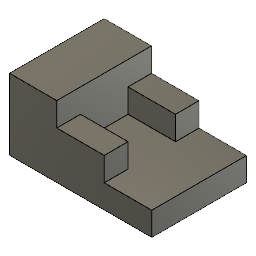
3DD6 (Autodesk Fusion 360 design; units mm, degrees)
Autodesk Fusion 360 part; units mm, degrees
sketch "Sketch1" plane through (0, 0, 0) normal (0, 1, 0) x (1, 0, 0)
  line L0 (0, 0) -> (60, 0)
  line L1 (60, 0) -> (60, -40)
  line L2 (60, -40) -> (0, -40)
  line L3 (0, -40) -> (0, 0)
  dimension "d1" = 60
  dimension "d2" = 40
  measures "d2" distance of L0.start
extrude "Extrude1" add sketch "Sketch1" along normal blind 10
sketch "Sketch2" plane through (0, 10, 0) normal (0, 1, 0) x (-1, 0, 0)
  line L0 (0, 40) -> (-60, 40)
  line L1 (-60, 40) -> (-60, 0)
  line L2 (-60, 0) -> (0, 0)
  line L3 (0, 0) -> (0, 40)
  line L4 (0, 0) -> (-20, 0)
  line L5 (-20, 0) -> (-20, 40)
  line L6 (-20, 40) -> (0, 40)
  line L7 (0, 40) -> (0, 0)
  dimension "d5" = 20
extrude "Extrude2" add sketch "Sketch2" along normal blind 20 contours L0 L2 L3 L4 L5 L6 L7
sketch "Sketch3" plane through (0, 10, 0) normal (0, 1, 0) x (-1, 0, 0)
  line L0 (-20, 0) -> (-20, 40)
  line L1 (-20, 40) -> (-60, 40)
  line L2 (-60, 40) -> (-60, 0)
  line L3 (-60, 0) -> (-20, 0)
  line L4 (-20, 0) -> (-40, 0)
  line L5 (-40, 0) -> (-40, 10)
  line L6 (-40, 10) -> (-20, 10)
  line L7 (-20, 10) -> (-20, 0)
  line L8 (-20, 40) -> (-40, 40)
  line L9 (-40, 40) -> (-40, 30)
  line L10 (-40, 30) -> (-20, 30)
  line L11 (-20, 30) -> (-20, 40)
  dimension "d8" = 20
  dimension "d9" = 20
  dimension "d10" = 10
  dimension "d11" = 10
  measures "d10" distance of origin
extrude "Extrude3" add sketch "Sketch3" along normal blind 10 contours L0 L3 L4 L5 L6 L7 | L0 L1 L8 L9 L10 L11
